kontentkelder2 (Autodesk Fusion 360 design; units mm, degrees)
Autodesk Fusion 360 part; units mm, degrees
sketch "Sketch1" plane through (0, 0, 0) normal (0, 1, 0) x (1, 0, 0)
  line L0 (0, 0) -> (-146, 0)
  line L1 (-146, 0) -> (-146, -41)
  line L2 (-146, -41) -> (0, -41)
  line L3 (0, -41) -> (0, 0)
  line L4 (-131.367, -21.2138) -> (-133.2967, -21.2138)
  line L5 (-133.2967, -21.2138) -> (-133.2967, -23.7241)
  line L6 (-133.2967, -23.7241) -> (-134.0655, -23.7241)
  line L7 (-134.0655, -23.7241) -> (-135.4383, -26.6971)
  spline S0 degree 2 poles (-135.4383, -26.6971) (-135.4696, -26.7599) (-135.5716, -26.9403) knots 0 0 0 1 1 1
  spline S1 degree 2 poles (-135.5716, -26.9403) (-135.6265, -27.0344) (-135.8619, -27.4816) knots 0 0 0 1 1 1
  spline S2 degree 2 poles (-135.8619, -27.4816) (-136.2541, -28.219) (-136.458, -28.4229) knots 0 0 0 1 1 1
  spline S3 degree 2 poles (-136.458, -28.4229) (-136.8032, -28.7524) (-137.47, -28.7602) knots 0 0 0 1 1 1
  line L8 (-137.47, -28.7602) -> (-137.47, -23.7241)
  line L9 (-137.47, -23.7241) -> (-139.792, -23.7241)
  line L10 (-139.792, -23.7241) -> (-139.792, -35.2241)
  line L11 (-139.792, -35.2241) -> (-137.47, -35.2241)
  line L12 (-137.47, -35.2241) -> (-137.47, -30.3291)
  spline S4 degree 2 poles (-137.47, -30.3291) (-136.5992, -30.4154) (-136.1835, -31.043) knots 0 0 0 1 1 1
  spline S5 degree 2 poles (-136.1835, -31.043) (-136.0815, -31.2156) (-135.5716, -32.5177) knots 0 0 0 1 1 1
  spline S6 degree 2 poles (-135.5716, -32.5177) (-134.9127, -34.22) (-134.2538, -34.7299) knots 0 0 0 1 1 1
  spline S7 degree 2 poles (-134.2538, -34.7299) (-133.5242, -35.2947) (-131.7906, -35.2947) knots 0 0 0 1 1 1
  spline S8 degree 2 poles (-131.7906, -35.2947) (-131.7121, -35.2947) (-131.4533, -35.3025) knots 0 0 0 1 1 1
  line L13 (-131.4533, -35.3025) -> (-131.4533, -33.5846)
  line L14 (-131.4533, -33.5846) -> (-131.7827, -33.5924)
  spline S9 degree 2 poles (-131.7827, -33.5924) (-132.9437, -33.6238) (-133.3595, -32.8786) knots 0 0 0 1 1 1
  spline S10 degree 2 poles (-133.3595, -32.8786) (-133.5634, -32.5177) (-133.9635, -31.396) knots 0 0 0 1 1 1
  spline S11 degree 2 poles (-133.9635, -31.396) (-134.2145, -30.69) (-134.442, -30.3762) knots 0 0 0 1 1 1
  spline S12 degree 2 poles (-134.442, -30.3762) (-134.7244, -29.9683) (-135.2971, -29.6467) knots 0 0 0 1 1 1
  spline S13 degree 2 poles (-135.2971, -29.6467) (-134.5126, -29.427) (-134.0106, -28.7602) knots 0 0 0 1 1 1
  spline S14 degree 2 poles (-134.0106, -28.7602) (-133.4458, -28.015) (-132.9045, -26.8776) knots 0 0 0 1 1 1
  line L15 (-132.9045, -26.8776) -> (-132.324, -25.6538)
  line L16 (-132.324, -25.6538) -> (-131.367, -25.6538)
  line L17 (-131.367, -25.6538) -> (-131.367, -21.2138)
  line L18 (-121.4751, -34.3847) -> (-120.2357, -35.7732)
  line L19 (-120.2357, -35.7732) -> (-119.1453, -34.8162)
  line L20 (-119.1453, -34.8162) -> (-120.4553, -33.3414)
  spline S15 degree 2 poles (-120.4553, -33.3414) (-119.9297, -32.6354) (-119.6395, -31.6039) knots 0 0 0 1 1 1
  spline S16 degree 2 poles (-119.6395, -31.6039) (-119.3492, -30.5723) (-119.3492, -29.4113) knots 0 0 0 1 1 1
  spline S17 degree 2 poles (-119.3492, -29.4113) (-119.3492, -26.6736) (-120.8632, -25.1008) knots 0 0 0 1 1 1
  spline S18 degree 2 poles (-120.8632, -25.1008) (-122.3772, -23.528) (-124.8639, -23.528) knots 0 0 0 1 1 1
  spline S19 degree 2 poles (-124.8639, -23.528) (-127.0211, -23.528) (-128.3155, -24.5085) knots 0 0 0 1 1 1
  line L21 (-128.3155, -24.5085) -> (-129.5863, -23.0808)
  line L22 (-129.5863, -23.0808) -> (-130.7002, -24.0535)
  line L23 (-130.7002, -24.0535) -> (-129.3588, -25.5597)
  spline S20 degree 2 poles (-129.3588, -25.5597) (-130.5041, -27.0894) (-130.5041, -29.5447) knots 0 0 0 1 1 1
  spline S21 degree 2 poles (-130.5041, -29.5447) (-130.5041, -32.2667) (-128.9901, -33.8435) knots 0 0 0 1 1 1
  spline S22 degree 2 poles (-128.9901, -33.8435) (-127.4761, -35.4202) (-124.9502, -35.4202) knots 0 0 0 1 1 1
  spline S23 degree 2 poles (-124.9502, -35.4202) (-122.8557, -35.4202) (-121.4751, -34.3847) knots 0 0 0 1 1 1
  spline S24 degree 2 poles (-122.9185, -32.7688) (-123.7108, -33.4434) (-124.9267, -33.4434) knots 0 0 0 1 1 1
  spline S25 degree 2 poles (-124.9267, -33.4434) (-126.3544, -33.4434) (-127.2329, -32.4589) knots 0 0 0 1 1 1
  spline S26 degree 2 poles (-127.2329, -32.4589) (-128.1115, -31.4744) (-128.1115, -29.4898) knots 0 0 0 1 1 1
  spline S27 degree 2 poles (-128.1115, -29.4898) (-128.1115, -28.2425) (-127.7507, -27.3561) knots 0 0 0 1 1 1
  line L24 (-127.7507, -27.3561) -> (-122.9185, -32.7688)
  line L25 (-122.0634, -31.5372) -> (-126.8878, -26.1166)
  spline S28 degree 2 poles (-126.8878, -26.1166) (-126.0798, -25.4106) (-124.9424, -25.4106) knots 0 0 0 1 1 1
  spline S29 degree 2 poles (-124.9424, -25.4106) (-123.546, -25.4106) (-122.6479, -26.4226) knots 0 0 0 1 1 1
  spline S30 degree 2 poles (-122.6479, -26.4226) (-121.7497, -27.4345) (-121.7497, -29.4427) knots 0 0 0 1 1 1
  spline S31 degree 2 poles (-121.7497, -29.4427) (-121.7497, -30.7135) (-122.0634, -31.5372) knots 0 0 0 1 1 1
  line L26 (-116.7057, -35.2241) -> (-108.6494, -35.2241)
  line L27 (-108.6494, -35.2241) -> (-108.6494, -23.7241)
  line L28 (-108.6494, -23.7241) -> (-110.9714, -23.7241)
  line L29 (-110.9714, -23.7241) -> (-110.9714, -33.2786)
  line L30 (-110.9714, -33.2786) -> (-114.4308, -33.2786)
  line L31 (-114.4308, -33.2786) -> (-114.4308, -28.368)
  spline S32 degree 2 poles (-114.4308, -28.368) (-114.4308, -26.2578) (-114.572, -25.4224) knots 0 0 0 1 1 1
  spline S33 degree 2 poles (-114.572, -25.4224) (-114.7132, -24.587) (-115.2584, -24.1202) knots 0 0 0 1 1 1
  spline S34 degree 2 poles (-115.2584, -24.1202) (-115.8035, -23.6535) (-116.9645, -23.6535) knots 0 0 0 1 1 1
  spline S35 degree 2 poles (-116.9645, -23.6535) (-117.3724, -23.6535) (-118.4471, -23.7319) knots 0 0 0 1 1 1
  line L32 (-118.4471, -23.7319) -> (-118.4471, -25.5283)
  line L33 (-118.4471, -25.5283) -> (-117.9294, -25.5205)
  spline S36 degree 2 poles (-117.9294, -25.5205) (-117.1999, -25.5205) (-116.9488, -25.7166) knots 0 0 0 1 1 1
  spline S37 degree 2 poles (-116.9488, -25.7166) (-116.6978, -25.9127) (-116.6978, -26.6814) knots 0 0 0 1 1 1
  line L34 (-116.6978, -26.6814) -> (-116.7057, -28.6583)
  line L35 (-116.7057, -28.6583) -> (-116.7057, -35.2241)
  line L36 (-103.6681, -23.7241) -> (-103.6681, -33.2786)
  line L37 (-103.6681, -33.2786) -> (-107.0805, -33.2786)
  line L38 (-107.0805, -33.2786) -> (-107.0805, -35.2241)
  line L39 (-107.0805, -35.2241) -> (-97.9417, -35.2241)
  line L40 (-97.9417, -35.2241) -> (-97.9417, -33.2786)
  line L41 (-97.9417, -33.2786) -> (-101.3462, -33.2786)
  line L42 (-101.3462, -33.2786) -> (-101.3462, -23.7241)
  line L43 (-101.3462, -23.7241) -> (-103.6681, -23.7241)
  line L44 (-105.2841, -38.2442) -> (-103.5034, -38.2442)
  line L45 (-103.5034, -38.2442) -> (-102.6562, -37.0754)
  line L46 (-102.6562, -37.0754) -> (-101.7463, -38.2442)
  line L47 (-101.7463, -38.2442) -> (-99.9734, -38.2442)
  line L48 (-99.9734, -38.2442) -> (-101.5972, -35.9301)
  line L49 (-101.5972, -35.9301) -> (-103.6368, -35.9301)
  line L50 (-103.6368, -35.9301) -> (-105.2841, -38.2442)
  spline S38 degree 2 poles (-87.8929, -26.3755) (-88.4106, -24.7517) (-89.5246, -24.1006) knots 0 0 0 1 1 1
  spline S39 degree 2 poles (-89.5246, -24.1006) (-90.4973, -23.528) (-92.3093, -23.528) knots 0 0 0 1 1 1
  spline S40 degree 2 poles (-92.3093, -23.528) (-94.1842, -23.528) (-95.3452, -24.2653) knots 0 0 0 1 1 1
  spline S41 degree 2 poles (-95.3452, -24.2653) (-96.7415, -25.1439) (-96.7415, -26.9089) knots 0 0 0 1 1 1
  spline S42 degree 2 poles (-96.7415, -26.9089) (-96.7415, -29.0034) (-94.4509, -29.7879) knots 0 0 0 1 1 1
  spline S43 degree 2 poles (-94.4509, -29.7879) (-96.3336, -30.792) (-96.3336, -32.4393) knots 0 0 0 1 1 1
  spline S44 degree 2 poles (-96.3336, -32.4393) (-96.3336, -33.9454) (-94.9765, -34.7534) knots 0 0 0 1 1 1
  spline S45 degree 2 poles (-94.9765, -34.7534) (-93.8547, -35.4202) (-92.2466, -35.4202) knots 0 0 0 1 1 1
  spline S46 degree 2 poles (-92.2466, -35.4202) (-88.8264, -35.4202) (-88.0969, -32.6119) knots 0 0 0 1 1 1
  line L51 (-88.0969, -32.6119) -> (-90.3561, -32.0863)
  spline S47 degree 2 poles (-90.3561, -32.0863) (-90.764, -33.5297) (-92.2231, -33.5297) knots 0 0 0 1 1 1
  spline S48 degree 2 poles (-92.2231, -33.5297) (-92.9683, -33.5297) (-93.4546, -33.161) knots 0 0 0 1 1 1
  spline S49 degree 2 poles (-93.4546, -33.161) (-93.9959, -32.7609) (-93.9959, -32.0392) knots 0 0 0 1 1 1
  spline S50 degree 2 poles (-93.9959, -32.0392) (-93.9959, -31.145) (-93.3213, -30.6821) knots 0 0 0 1 1 1
  spline S51 degree 2 poles (-93.3213, -30.6821) (-92.7408, -30.2899) (-91.7995, -30.2899) knots 0 0 0 1 1 1
  line L52 (-91.7995, -30.2899) -> (-91.5327, -30.2899)
  line L53 (-91.5327, -30.2899) -> (-91.5327, -28.5563)
  line L54 (-91.5327, -28.5563) -> (-92.0583, -28.5563)
  spline S52 degree 2 poles (-92.0583, -28.5563) (-92.9918, -28.5563) (-93.5801, -28.2425) knots 0 0 0 1 1 1
  spline S53 degree 2 poles (-93.5801, -28.2425) (-94.3411, -27.8346) (-94.3411, -26.9874) knots 0 0 0 1 1 1
  spline S54 degree 2 poles (-94.3411, -26.9874) (-94.3411, -26.1872) (-93.6586, -25.7715) knots 0 0 0 1 1 1
  spline S55 degree 2 poles (-93.6586, -25.7715) (-93.0859, -25.4263) (-92.2387, -25.4263) knots 0 0 0 1 1 1
  spline S56 degree 2 poles (-92.2387, -25.4263) (-91.2974, -25.4263) (-90.8032, -25.795) knots 0 0 0 1 1 1
  spline S57 degree 2 poles (-90.8032, -25.795) (-90.309, -26.1637) (-90.0188, -27.0737) knots 0 0 0 1 1 1
  line L55 (-90.0188, -27.0737) -> (-87.8929, -26.3755)
  line L56 (-85.5553, -35.2241) -> (-77.499, -35.2241)
  line L57 (-77.499, -35.2241) -> (-77.499, -23.7241)
  line L58 (-77.499, -23.7241) -> (-79.8209, -23.7241)
  line L59 (-79.8209, -23.7241) -> (-79.8209, -33.2786)
  line L60 (-79.8209, -33.2786) -> (-83.2804, -33.2786)
  line L61 (-83.2804, -33.2786) -> (-83.2804, -28.368)
  spline S58 degree 2 poles (-83.2804, -28.368) (-83.2804, -26.2578) (-83.4216, -25.4224) knots 0 0 0 1 1 1
  spline S59 degree 2 poles (-83.4216, -25.4224) (-83.5628, -24.587) (-84.108, -24.1202) knots 0 0 0 1 1 1
  spline S60 degree 2 poles (-84.108, -24.1202) (-84.6531, -23.6535) (-85.8141, -23.6535) knots 0 0 0 1 1 1
  spline S61 degree 2 poles (-85.8141, -23.6535) (-86.222, -23.6535) (-87.2967, -23.7319) knots 0 0 0 1 1 1
  line L62 (-87.2967, -23.7319) -> (-87.2967, -25.5283)
  line L63 (-87.2967, -25.5283) -> (-86.779, -25.5205)
  spline S62 degree 2 poles (-86.779, -25.5205) (-86.0495, -25.5205) (-85.7984, -25.7166) knots 0 0 0 1 1 1
  spline S63 degree 2 poles (-85.7984, -25.7166) (-85.5474, -25.9127) (-85.5474, -26.6814) knots 0 0 0 1 1 1
  line L64 (-85.5474, -26.6814) -> (-85.5553, -28.6583)
  line L65 (-85.5553, -28.6583) -> (-85.5553, -35.2241)
  line L66 (-72.5177, -23.7241) -> (-72.5177, -33.2786)
  line L67 (-72.5177, -33.2786) -> (-75.9301, -33.2786)
  line L68 (-75.9301, -33.2786) -> (-75.9301, -35.2241)
  line L69 (-75.9301, -35.2241) -> (-66.7913, -35.2241)
  line L70 (-66.7913, -35.2241) -> (-66.7913, -33.2786)
  line L71 (-66.7913, -33.2786) -> (-70.1958, -33.2786)
  line L72 (-70.1958, -33.2786) -> (-70.1958, -23.7241)
  line L73 (-70.1958, -23.7241) -> (-72.5177, -23.7241)
  line L74 (-74.1337, -38.2442) -> (-72.353, -38.2442)
  line L75 (-72.353, -38.2442) -> (-71.5058, -37.0754)
  line L76 (-71.5058, -37.0754) -> (-70.5958, -38.2442)
  line L77 (-70.5958, -38.2442) -> (-68.823, -38.2442)
  line L78 (-68.823, -38.2442) -> (-70.4468, -35.9301)
  line L79 (-70.4468, -35.9301) -> (-72.4864, -35.9301)
  line L80 (-72.4864, -35.9301) -> (-74.1337, -38.2442)
  line L81 (-64.4144, -3.2657) -> (-66.3441, -3.2657)
  line L82 (-66.3441, -3.2657) -> (-66.3441, -5.7759)
  line L83 (-66.3441, -5.7759) -> (-67.1129, -5.7759)
  line L84 (-67.1129, -5.7759) -> (-68.4857, -8.749)
  spline S64 degree 2 poles (-68.4857, -8.749) (-68.5171, -8.8117) (-68.619, -8.9922) knots 0 0 0 1 1 1
  spline S65 degree 2 poles (-68.619, -8.9922) (-68.6739, -9.0863) (-68.9093, -9.5334) knots 0 0 0 1 1 1
  spline S66 degree 2 poles (-68.9093, -9.5334) (-69.3015, -10.2708) (-69.5055, -10.4748) knots 0 0 0 1 1 1
  spline S67 degree 2 poles (-69.5055, -10.4748) (-69.8506, -10.8042) (-70.5174, -10.8121) knots 0 0 0 1 1 1
  line L85 (-70.5174, -10.8121) -> (-70.5174, -5.7759)
  line L86 (-70.5174, -5.7759) -> (-72.8394, -5.7759)
  line L87 (-72.8394, -5.7759) -> (-72.8394, -17.2759)
  line L88 (-72.8394, -17.2759) -> (-70.5174, -17.2759)
  line L89 (-70.5174, -17.2759) -> (-70.5174, -12.381)
  spline S68 degree 2 poles (-70.5174, -12.381) (-69.6467, -12.4673) (-69.2309, -13.0948) knots 0 0 0 1 1 1
  spline S69 degree 2 poles (-69.2309, -13.0948) (-69.1289, -13.2674) (-68.619, -14.5696) knots 0 0 0 1 1 1
  spline S70 degree 2 poles (-68.619, -14.5696) (-67.9601, -16.2718) (-67.3012, -16.7817) knots 0 0 0 1 1 1
  spline S71 degree 2 poles (-67.3012, -16.7817) (-66.5716, -17.3465) (-64.838, -17.3465) knots 0 0 0 1 1 1
  spline S72 degree 2 poles (-64.838, -17.3465) (-64.7596, -17.3465) (-64.5007, -17.3544) knots 0 0 0 1 1 1
  line L90 (-64.5007, -17.3544) -> (-64.5007, -15.6364)
  line L91 (-64.5007, -15.6364) -> (-64.8302, -15.6443)
  spline S73 degree 2 poles (-64.8302, -15.6443) (-65.9911, -15.6756) (-66.4069, -14.9304) knots 0 0 0 1 1 1
  spline S74 degree 2 poles (-66.4069, -14.9304) (-66.6108, -14.5696) (-67.0109, -13.4478) knots 0 0 0 1 1 1
  spline S75 degree 2 poles (-67.0109, -13.4478) (-67.2619, -12.7418) (-67.4894, -12.428) knots 0 0 0 1 1 1
  spline S76 degree 2 poles (-67.4894, -12.428) (-67.7718, -12.0201) (-68.3445, -11.6985) knots 0 0 0 1 1 1
  spline S77 degree 2 poles (-68.3445, -11.6985) (-67.56, -11.4789) (-67.058, -10.8121) knots 0 0 0 1 1 1
  spline S78 degree 2 poles (-67.058, -10.8121) (-66.4932, -10.0668) (-65.9519, -8.9294) knots 0 0 0 1 1 1
  line L92 (-65.9519, -8.9294) -> (-65.3714, -7.7057)
  line L93 (-65.3714, -7.7057) -> (-64.4144, -7.7057)
  line L94 (-64.4144, -7.7057) -> (-64.4144, -3.2657)
  spline S79 degree 2 poles (-54.5225, -8.4274) (-55.0402, -6.8035) (-56.1542, -6.1525) knots 0 0 0 1 1 1
  spline S80 degree 2 poles (-56.1542, -6.1525) (-57.1269, -5.5798) (-58.9389, -5.5798) knots 0 0 0 1 1 1
  spline S81 degree 2 poles (-58.9389, -5.5798) (-60.8138, -5.5798) (-61.9748, -6.3172) knots 0 0 0 1 1 1
  spline S82 degree 2 poles (-61.9748, -6.3172) (-63.3711, -7.1958) (-63.3711, -8.9608) knots 0 0 0 1 1 1
  spline S83 degree 2 poles (-63.3711, -8.9608) (-63.3711, -11.0553) (-61.0805, -11.8397) knots 0 0 0 1 1 1
  spline S84 degree 2 poles (-61.0805, -11.8397) (-62.9632, -12.8438) (-62.9632, -14.4911) knots 0 0 0 1 1 1
  spline S85 degree 2 poles (-62.9632, -14.4911) (-62.9632, -15.9973) (-61.6061, -16.8053) knots 0 0 0 1 1 1
  spline S86 degree 2 poles (-61.6061, -16.8053) (-60.4843, -17.472) (-58.8762, -17.472) knots 0 0 0 1 1 1
  spline S87 degree 2 poles (-58.8762, -17.472) (-55.456, -17.472) (-54.7265, -14.6637) knots 0 0 0 1 1 1
  line L95 (-54.7265, -14.6637) -> (-56.9857, -14.1381)
  spline S88 degree 2 poles (-56.9857, -14.1381) (-57.3936, -15.5815) (-58.8527, -15.5815) knots 0 0 0 1 1 1
  spline S89 degree 2 poles (-58.8527, -15.5815) (-59.5979, -15.5815) (-60.0842, -15.2128) knots 0 0 0 1 1 1
  spline S90 degree 2 poles (-60.0842, -15.2128) (-60.6255, -14.8128) (-60.6255, -14.0911) knots 0 0 0 1 1 1
  spline S91 degree 2 poles (-60.6255, -14.0911) (-60.6255, -13.1968) (-59.9509, -12.734) knots 0 0 0 1 1 1
  spline S92 degree 2 poles (-59.9509, -12.734) (-59.3704, -12.3417) (-58.4291, -12.3417) knots 0 0 0 1 1 1
  line L96 (-58.4291, -12.3417) -> (-58.1623, -12.3417)
  line L97 (-58.1623, -12.3417) -> (-58.1623, -10.6081)
  line L98 (-58.1623, -10.6081) -> (-58.6879, -10.6081)
  spline S93 degree 2 poles (-58.6879, -10.6081) (-59.6214, -10.6081) (-60.2098, -10.2943) knots 0 0 0 1 1 1
  spline S94 degree 2 poles (-60.2098, -10.2943) (-60.9707, -9.8864) (-60.9707, -9.0392) knots 0 0 0 1 1 1
  spline S95 degree 2 poles (-60.9707, -9.0392) (-60.9707, -8.2391) (-60.2882, -7.8233) knots 0 0 0 1 1 1
  spline S96 degree 2 poles (-60.2882, -7.8233) (-59.7156, -7.4782) (-58.8683, -7.4782) knots 0 0 0 1 1 1
  spline S97 degree 2 poles (-58.8683, -7.4782) (-57.927, -7.4782) (-57.4328, -7.8469) knots 0 0 0 1 1 1
  spline S98 degree 2 poles (-57.4328, -7.8469) (-56.9386, -8.2156) (-56.6484, -9.1255) knots 0 0 0 1 1 1
  line L99 (-56.6484, -9.1255) -> (-54.5225, -8.4274)
  line L100 (-52.883, -11.5181) -> (-52.883, -17.2759)
  line L101 (-52.883, -17.2759) -> (-50.5689, -17.2759)
  line L102 (-50.5689, -17.2759) -> (-50.5689, -13.4714)
  line L103 (-50.5689, -13.4714) -> (-47.9881, -15.6364)
  line L104 (-47.9881, -15.6364) -> (-47.9881, -13.7381)
  line L105 (-47.9881, -13.7381) -> (-50.5689, -11.5808)
  line L106 (-50.5689, -11.5808) -> (-50.5689, -7.7135)
  line L107 (-50.5689, -7.7135) -> (-44.7875, -7.7135)
  line L108 (-44.7875, -7.7135) -> (-44.7875, -5.7759)
  line L109 (-44.7875, -5.7759) -> (-52.883, -5.7759)
  line L110 (-52.883, -5.7759) -> (-52.883, -9.6511)
  line L111 (-52.883, -9.6511) -> (-54.0989, -8.6392)
  line L112 (-54.0989, -8.6392) -> (-54.0989, -10.4983)
  line L113 (-54.0989, -10.4983) -> (-52.883, -11.5181)
  line L114 (-43.1951, -17.2759) -> (-38.9591, -17.2759)
  spline S99 degree 2 poles (-38.9591, -17.2759) (-37.5, -17.2759) (-36.7469, -17.0484) knots 0 0 0 1 1 1
  spline S100 degree 2 poles (-36.7469, -17.0484) (-35.7272, -16.7425) (-35.0055, -15.9698) knots 0 0 0 1 1 1
  spline S101 degree 2 poles (-35.0055, -15.9698) (-34.2838, -15.1971) (-33.919, -14.0989) knots 0 0 0 1 1 1
  spline S102 degree 2 poles (-33.919, -14.0989) (-33.5542, -13.0007) (-33.5542, -11.3847) knots 0 0 0 1 1 1
  spline S103 degree 2 poles (-33.5542, -11.3847) (-33.5542, -9.9649) (-33.9582, -8.8235) knots 0 0 0 1 1 1
  spline S104 degree 2 poles (-33.9582, -8.8235) (-34.3622, -7.6821) (-35.1467, -6.9212) knots 0 0 0 1 1 1
  spline S105 degree 2 poles (-35.1467, -6.9212) (-35.7507, -6.3486) (-36.7705, -6.0191) knots 0 0 0 1 1 1
  spline S106 degree 2 poles (-36.7705, -6.0191) (-37.5392, -5.7759) (-38.8336, -5.7759) knots 0 0 0 1 1 1
  line L115 (-38.8336, -5.7759) -> (-43.1951, -5.7759)
  line L116 (-43.1951, -5.7759) -> (-43.1951, -10.7964)
  line L117 (-43.1951, -10.7964) -> (-44.3875, -10.7964)
  line L118 (-44.3875, -10.7964) -> (-44.3875, -12.2555)
  line L119 (-44.3875, -12.2555) -> (-43.1951, -12.2555)
  line L120 (-43.1951, -12.2555) -> (-43.1951, -17.2759)
  line L121 (-40.881, -15.3305) -> (-40.881, -12.2555)
  line L122 (-40.881, -12.2555) -> (-38.4178, -12.2555)
  line L123 (-38.4178, -12.2555) -> (-38.4178, -10.7964)
  line L124 (-38.4178, -10.7964) -> (-40.881, -10.7964)
  line L125 (-40.881, -10.7964) -> (-40.881, -7.7135)
  line L126 (-40.881, -7.7135) -> (-39.1395, -7.7135)
  spline S107 degree 2 poles (-39.1395, -7.7135) (-37.9864, -7.7135) (-37.4765, -7.9018) knots 0 0 0 1 1 1
  spline S108 degree 2 poles (-37.4765, -7.9018) (-36.8018, -8.1371) (-36.4488, -8.7647) knots 0 0 0 1 1 1
  spline S109 degree 2 poles (-36.4488, -8.7647) (-35.9546, -9.6511) (-35.9546, -11.471) knots 0 0 0 1 1 1
  spline S110 degree 2 poles (-35.9546, -11.471) (-35.9546, -12.7653) (-36.1625, -13.4674) knots 0 0 0 1 1 1
  spline S111 degree 2 poles (-36.1625, -13.4674) (-36.3704, -14.1695) (-36.7744, -14.601) knots 0 0 0 1 1 1
  spline S112 degree 2 poles (-36.7744, -14.601) (-37.1784, -15.0324) (-37.8295, -15.205) knots 0 0 0 1 1 1
  spline S113 degree 2 poles (-37.8295, -15.205) (-38.3315, -15.3305) (-39.8298, -15.3305) knots 0 0 0 1 1 1
  line L127 (-39.8298, -15.3305) -> (-40.881, -15.3305)
  spline S114 degree 2 poles (-23.0426, -8.4274) (-23.5604, -6.8035) (-24.6743, -6.1525) knots 0 0 0 1 1 1
  spline S115 degree 2 poles (-24.6743, -6.1525) (-25.647, -5.5798) (-27.4591, -5.5798) knots 0 0 0 1 1 1
  spline S116 degree 2 poles (-27.4591, -5.5798) (-29.3339, -5.5798) (-30.4949, -6.3172) knots 0 0 0 1 1 1
  spline S117 degree 2 poles (-30.4949, -6.3172) (-31.8912, -7.1958) (-31.8912, -8.9608) knots 0 0 0 1 1 1
  spline S118 degree 2 poles (-31.8912, -8.9608) (-31.8912, -11.0553) (-29.6006, -11.8397) knots 0 0 0 1 1 1
  spline S119 degree 2 poles (-29.6006, -11.8397) (-31.4833, -12.8438) (-31.4833, -14.4911) knots 0 0 0 1 1 1
  spline S120 degree 2 poles (-31.4833, -14.4911) (-31.4833, -15.9973) (-30.1262, -16.8053) knots 0 0 0 1 1 1
  spline S121 degree 2 poles (-30.1262, -16.8053) (-29.0044, -17.472) (-27.3963, -17.472) knots 0 0 0 1 1 1
  spline S122 degree 2 poles (-27.3963, -17.472) (-23.9761, -17.472) (-23.2466, -14.6637) knots 0 0 0 1 1 1
  line L128 (-23.2466, -14.6637) -> (-25.5058, -14.1381)
  spline S123 degree 2 poles (-25.5058, -14.1381) (-25.9137, -15.5815) (-27.3728, -15.5815) knots 0 0 0 1 1 1
  spline S124 degree 2 poles (-27.3728, -15.5815) (-28.118, -15.5815) (-28.6044, -15.2128) knots 0 0 0 1 1 1
  spline S125 degree 2 poles (-28.6044, -15.2128) (-29.1456, -14.8128) (-29.1456, -14.0911) knots 0 0 0 1 1 1
  spline S126 degree 2 poles (-29.1456, -14.0911) (-29.1456, -13.1968) (-28.471, -12.734) knots 0 0 0 1 1 1
  spline S127 degree 2 poles (-28.471, -12.734) (-27.8905, -12.3417) (-26.9492, -12.3417) knots 0 0 0 1 1 1
  line L129 (-26.9492, -12.3417) -> (-26.6825, -12.3417)
  line L130 (-26.6825, -12.3417) -> (-26.6825, -10.6081)
  line L131 (-26.6825, -10.6081) -> (-27.2081, -10.6081)
  spline S128 degree 2 poles (-27.2081, -10.6081) (-28.1416, -10.6081) (-28.7299, -10.2943) knots 0 0 0 1 1 1
  spline S129 degree 2 poles (-28.7299, -10.2943) (-29.4908, -9.8864) (-29.4908, -9.0392) knots 0 0 0 1 1 1
  spline S130 degree 2 poles (-29.4908, -9.0392) (-29.4908, -8.2391) (-28.8083, -7.8233) knots 0 0 0 1 1 1
  spline S131 degree 2 poles (-28.8083, -7.8233) (-28.2357, -7.4782) (-27.3885, -7.4782) knots 0 0 0 1 1 1
  spline S132 degree 2 poles (-27.3885, -7.4782) (-26.4471, -7.4782) (-25.9529, -7.8469) knots 0 0 0 1 1 1
  spline S133 degree 2 poles (-25.9529, -7.8469) (-25.4587, -8.2156) (-25.1685, -9.1255) knots 0 0 0 1 1 1
  line L132 (-25.1685, -9.1255) -> (-23.0426, -8.4274)
  line L133 (-14.8589, -11.9633) -> (-17.829, -11.9633)
  line L134 (-17.829, -11.9633) -> (-17.829, -11.2563)
  spline S134 degree 2 poles (-17.829, -11.2563) (-17.829, -7.4919) (-20.6501, -4.361) knots 0 0 0 1 1 1
  line L135 (-20.6501, -4.361) -> (-22.0209, -5.6328)
  spline S135 degree 2 poles (-22.0209, -5.6328) (-19.7107, -7.9077) (-19.7107, -12.1172) knots 0 0 0 1 1 1
  line L136 (-19.7107, -12.1172) -> (-19.7107, -17.9035)
  line L137 (-19.7107, -17.9035) -> (-9.0922, -17.9035)
  line L138 (-9.0922, -17.9035) -> (-9.0922, -11.4367)
  line L139 (-9.0922, -11.4367) -> (-10.9739, -11.4367)
  line L140 (-10.9739, -11.4367) -> (-10.9739, -11.9633)
  line L141 (-10.9739, -11.9633) -> (-13.2145, -11.9633)
  line L142 (-13.2145, -11.9633) -> (-13.1027, -11.6191)
  spline S136 degree 2 poles (-13.1027, -11.6191) (-12.4928, -8.2577) (-7.4919, -6.5202) knots 0 0 0 1 1 1
  line L143 (-7.4919, -6.5202) -> (-8.0548, -4.7297)
  spline S137 degree 2 poles (-8.0548, -4.7297) (-14.1911, -6.8075) (-14.8216, -11.7201) knots 0 0 0 1 1 1
  line L144 (-14.8216, -11.7201) -> (-14.8589, -11.9633)
  line L145 (-10.9739, -13.7194) -> (-10.9739, -16.1473)
  line L146 (-10.9739, -16.1473) -> (-17.829, -16.1473)
  line L147 (-17.829, -16.1473) -> (-17.829, -13.7194)
  line L148 (-17.829, -13.7194) -> (-10.9739, -13.7194)
  dimension "d1" = 146
  dimension "d2" = 41
  constraint horizontal L0
  constraint vertical L1
  constraint horizontal L2
  constraint vertical L3
  constraint coincident L0.start L3.end
  measures "d1" distance of L1.end L2.end
  measures "d2" distance of L0.start L2.end
extrude "Extrude1" add sketch "Sketch1" against normal blind 10 makes body 1 at (-13.2589, -3.3333, 16.1473) makes body 2 at (-40.881, -3.3333, 9.7688) makes body 3 at (-123.6716, -3.3333, 29.7303) makes body 4 at (-109.1629, 0, 9.8333) makes body 5 at (-126.1399, -3.3333, 29.1603)
extrude "Extrude2" add sketch "Sketch1" against normal blind 10 separate body contours L4 L5 L6 L7 S0 S1 S2 S3 L8 L9 L10 L11 L12 S4 S5 S6 S7 S8 L13 L14 S9 S10 S11 S12 S13 S14 L15 L16 L17 | L18 L19 L20 S15 S16 S17 S18 S19 L21 L22 L23 S20 S21 S22 S23 | L26 L27 L28 L29 L30 L31 S32 S33 S34 S35 L32 L33 S36 S37 L34 L35 | L36 L37 L38 L39 L40 L41 L42 L43 | L44 L45 L46 L47 L48 L49 L50 | S38 S39 S40 S41 S42 S43 S44 S45 S46 L51 S47 S48 S49 S50 S51 L52 L53 L54 S52 S53 S54 S55 S56 S57 L55 | L56 L57 L58 L59 L60 L61 S58 S59 S60 S61 L62 L63 S62 S63 L64 L65 | L66 L67 L68 L69 L70 L71 L72 L73 | L74 L75 L76 L77 L78 L79 L80 | L81 L82 L83 L84 S64 S65 S66 S67 L85 L86 L87 L88 L89 S68 S69 S70 S71 S72 L90 L91 S73 S74 S75 S76 S77 S78 L92 L93 L94 | S79 S80 S81 S82 S83 S84 S85 S86 S87 L95 S88 S89 S90 S91 S92 L96 L97 L98 S93 S94 S95 S96 S97 S98 L99 | L100 L101 L102 L103 L104 L105 L106 L107 L108 L109 L110 L111 L112 L113 | L114 S99 S100 S101 S102 S103 S104 S105 S106 L115 L116 L117 L118 L119 L120 | S114 S115 S116 S117 S118 S119 S120 S121 S122 L128 S123 S124 S125 S126 S127 L129 L130 L131 S128 S129 S130 S131 S132 S133 L132 | L133 L134 S134 L135 S135 L136 L137 L138 L139 L140 L141 L142 S136 L143 S137 L144 makes body 6 at (-42.4237, 0, 14.954) makes body 7 at (-104.1859, -3.3333, 36.7015) makes body 8 at (-91.6952, -4.1667, 35.4007) makes body 9 at (-139.792, -3.3333, 27.5574) makes body 10 at (-101.3462, -3.3333, 30.0938) makes body 11 at (-73.0355, -3.3333, 36.7015) makes body 12 at (-47.486, -3.3333, 5.7759) makes body 13 at (-26.845, -4.1667, 17.4525) makes body 14 at (-72.8394, -3.3333, 9.6093) makes body 15 at (-77.499, -3.3333, 31.3907) makes body 16 at (-125.8523, 0, 28.7472) makes body 17 at (-108.6494, -3.3333, 31.3907) makes body 18 at (-70.1958, -3.3333, 30.0938) makes body 19 at (-58.3248, -4.1667, 17.4525) makes body 20 at (-16.1712, -3.3333, 17.9035)
sketch "Sketch2" plane through (-73, 0, 20.5) normal (0, 1, 0) x (1, 0, 0)
  line L0 (65, -15.5) -> (-65, -15.5)
  line L1 (-65, -15.5) -> (-65, 15.5)
  line L2 (-65, 15.5) -> (65, 15.5)
  line L3 (65, 15.5) -> (65, -15.5)
  line L4 (-73, 20.5) -> (-73, -20.5)
  line L5 (73, -20.5) -> (73, 20.5)
  line L6 (-73, -20.5) -> (73, -20.5)
  line L7 (73, 20.5) -> (-73, 20.5)
  dimension "d12" = 8
  dimension "d13" = 8
  dimension "d14" = 5
  dimension "d15" = 5
  constraint horizontal L0
  constraint vertical L1
  constraint horizontal L2
  constraint vertical L3
  measures "d12" distance of L1 L4
  measures "d13" distance of L3 L5
  measures "d14" distance of L0 L6
  measures "d15" distance of L2 L7
extrude "Extrude3" add sketch "Sketch2" along normal blind 70 separate body makes body 21
combine "Combine1" operation add target body 4 tool bodies 21
copy_body "Body->Comp1" bodies 4 removing the originals makes body 22 in component "Component"
copy_body "CutPasteBodies1" bodies 1 2 3 5 removing the originals makes body 23 makes body 24 makes body 25 makes body 26 in component "Component"
copy_body "Body->Comp2" bodies 6 removing the originals makes body 27 in component "Component'"
copy_body "CutPasteBodies1'" bodies 8 14 20 10 12 16 13 18 9 15 19 7 17 11 removing the originals makes body 28 makes body 29 makes body 30 makes body 31 makes body 32 makes body 33 makes body 34 makes body 35 makes body 36 makes body 37 makes body 38 makes body 39 makes body 40 makes body 41 in component "Component'"
component "Component" placed x (1, 0, 0) y (0, 1, 0) z (0, 0, 1) at (0, 0, 0)
component "Component'" placed x (1, 0, 0) y (0, 1, 0) z (0, 0, 1) at (0, 0, 0)
equation "d13 = d12"
equation "d15 = d14"
